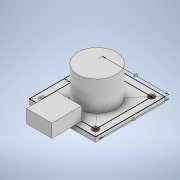
# Autodesk Inventor part: buzzer_footprint
Saved by Autodesk Inventor 2021 (Build 250183000, 183)
## iProperties
Created: 2021-12-12
Part Number: buzzer_footprint
Material: Generic
Document SubType Name: Modeling
Designer: Juan M. Casillas
Density: 1 g/cm^3
Appearance: Default
Author: Juan M. Casillas
Autodesk Inventor part; units mm, degrees
ref_plane "YZ Plane" through (0, 0, 0) normal (1, 0, 0) x (0, 1, 0)
ref_plane "XZ Plane" through (0, 0, 0) normal (0, 1, 0) x (-1, 0, 0)
ref_plane "XY Plane" through (0, 0, 0) normal (0, 0, 1) x (1, 0, 0)
sketch "Sketch1" plane through (0, 0, 0) normal (0, 1, 0) x (-1, 0, 0)
  line L0 (10, 10.5) -> (-10, 10.5)
  line L1 (-10, 10.5) -> (-10, -10.5)
  line L2 (-10, -10.5) -> (10, -10.5)
  line L3 (10, -10.5) -> (10, 10.5)
  line L4 (10, 10.5) -> (-10, -10.5) construction
  line L5 (-10, 10.5) -> (10, -10.5) construction
  line L6 (8, 8.5) -> (-8, 8.5)
  line L7 (-8, 8.5) -> (-8, -8.5)
  line L8 (-8, -8.5) -> (8, -8.5)
  line L9 (8, -8.5) -> (8, 8.5)
  point P0 (0, 0)
  dimension "d0" = 20
  dimension "d1" = 21
  dimension "d2" = 2
  constraints: 20 end point, 4 coincident, 4 parallel, 2 midpoint, 2 perpendicular, 1 horizontal, 3 other
  measures "d0" distance of L2.end L1.end
  measures "d1" distance of L1.end L0.end
  measures "d2" distance between parallel lines of L3 L9
extrude "Extrusion1" add sketch "Sketch1" against normal blind 1.5 contours L3 L2 L1 L0 | L9 L8 L7 L6
hole "Hole1" at (-8, 0, 8.5) at (-8, 0, -8.5) at (8, 0, -8.5) at (8, 0, 8.5) direction (0, -1, 0) diameter 2 end through all
sketch "Sketch2" plane through (0, 0, 0) normal (0, 1, 0) x (1, 0, 0)
  line L0 (-3.85, -8.5124) -> (3.85, -8.5124)
  line L1 (3.85, -8.5124) -> (3.85, -17.5124)
  line L2 (3.85, -17.5124) -> (-3.85, -17.5124)
  line L3 (-3.85, -17.5124) -> (-3.85, -8.5124)
  line L4 (-3.85, -8.5124) -> (3.85, -17.5124) construction
  line L5 (3.85, -8.5124) -> (-3.85, -17.5124) construction
  line L6 (-10, -10.5) -> (10, -10.5) projected
  line L7 (-10, 10.5) -> (-10, -10.5) projected
  point P0 (0, 0)
  point P1 (0, -13.0124)
  point P2 (0, -8.5124)
  point P3 (0, -8.5124)
  dimension "d12" = 7.7
  dimension "d13" = 9
  dimension "d14" = 1.9876
  dimension "d15" = 10
  constraints: 12 end point, 3 midpoint, 2 parallel, 1 coincident, 1 horizontal, 1 perpendicular
  measures "d12" distance of L1.end L2.end
  measures "d13" distance of L0.end L1.end
  measures "d14" distance from line of L6 point (0, -8.512)
  measures "d15" distance from line of L7 point (0, -8.512)
extrude "Extrusion2" add sketch "Sketch2" along normal blind 4
sketch "Sketch3" plane through (0, 0, 0) normal (0, 1, 0) x (1, 0, 0)
  circle A0 centre (0, 0) radius 5.85
  dimension "d18" = 11.7
  constraints: 1 centre point, 1 coincident
  measures "d18" diameter of A0
extrude "Extrusion3" add sketch "Sketch3" along normal blind 9
body "Solid1"
